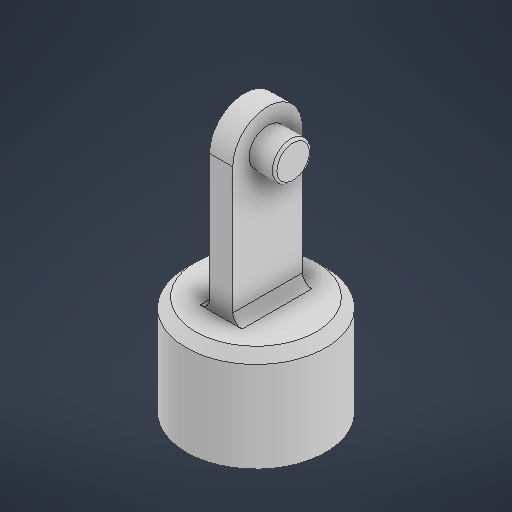
# Autodesk Inventor part: Peça3
Saved by Autodesk Inventor 2027 (Build 310192060, 192F)
## iProperties
Created: 2026-08-25
Part Number: Peça3
Material: Genérico
Document SubType Name: Modeling
Designer: guisg
Density: 1 g/cm^3
Appearance: Padrão
Author: guisg
Autodesk Inventor part; units mm, degrees
ref_plane "YZ Plane" through (0, 0, 0) normal (1, 0, 0) x (0, 1, 0)
ref_plane "XZ Plane" through (0, 0, 0) normal (0, 1, 0) x (-1, 0, 0)
ref_plane "XY Plane" through (0, 0, 0) normal (0, 0, 1) x (1, 0, 0)
sketch "Esboço1" plane through (0, 0, 0) normal (1, 0, 0) x (0, 1, 0)
  line L0 (0, 5) -> (10, 5)
  line L1 (10, 5) -> (10, -5)
  line L2 (10, -5) -> (0, -5)
  line L3 (0, 5) -> (0, 15)
  line L4 (0, -5) -> (0, -15)
  line L5 (0, 15) -> (21.5, 15)
  line L6 (21.5, 15) -> (21.5, -15)
  line L7 (21.5, -15) -> (0, -15)
  line L8 (0, 0) -> (50.75, 0)
  point P0 (21.5, 0)
  point P1 (10, 0)
  dimension "d8" = 50.75
  constraints: 18 end point, 3 perpendicular, 2 horizontal, 2 vertical
  measures "d8" distance of L8.start L8.end
revolve "Revolução1" add sketch "Esboço1" angle 360 mid plane about axis through (0, 0, 0) along (0, 1, 0) contours L8 L6 L7 L4 L2 L1
chamfer "Chanfro1" distance 2 angle 45 1 edges at (0, 21.5, -15) measured on face at (-1.207, 7.1667, 14.9514)
sketch "Esboço2" plane through (0, 0, 0) normal (1, 0, 0) x (0, 1, 0)
  line L0 (0, 0) -> (50.75, 0)
  circle A0 centre (50.75, 0) radius 4
  arc A1 (50.75, -7.5) -> (50.75, 7.5) centre (50.75, 0) ccw
  line L1 (50.75, 7.5) -> (21.5, 7.5)
  line L2 (50.75, -7.5) -> (21.5, -7.5)
  line L3 (21.5, 7.5) -> (21.5, -7.5)
  line L4 (21.5, 13) -> (21.5, -13) projected
  constraints: 8 end point, 2 centre point, 2 coincident, 2 horizontal, 2 point on circle, 1 collinear, 1 parallel, 1 tangent
extrude "Extrusão1" add sketch "Esboço2" along normal mid plane 5
fillet "Arredondamento1" radius 2 2 edges at (2.5, 21.5, 0) (-2.5, 21.5, 0)
sketch "Esboço3" plane through (2.5, 0, 0) normal (1, 0, 0) x (0, 0, -1)
  circle A0 centre (0, 50.75) radius 4 projected
  circle A1 centre (0, 50.75) radius 4
  point P0 (0, 0)
  dimension "d19" = 8
  constraints: 1 centre point, 1 coincident
  measures "d19" diameter of A1
extrude "Extrusão2" add sketch "Esboço3" along normal blind 5.5
fillet "Arredondamento2" radius 0.5 1 edges at (8, 50.75, 4)
